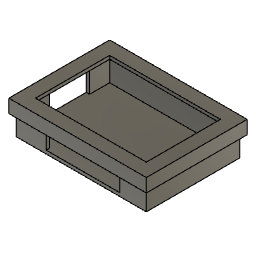
PCB box (Autodesk Fusion 360 design; units mm, degrees)
Autodesk Fusion 360 part; units mm, degrees
note: some values were not read from the file. Set by a fixed rule: which face or edge a step refers to.
sketch "Sketch1" plane through (0, 0, 0) normal (0, 0, 1) x (1, 0, 0) in component "base"
  line L0 (0, 0) -> (37, 0)
  line L1 (37, 0) -> (37, 26)
  line L2 (37, 26) -> (0, 26)
  line L3 (0, 26) -> (0, 0)
  dimension "d1" = 26
  dimension "d2" = 37
  constraint horizontal L0
  constraint vertical L1
  constraint horizontal L2
  constraint vertical L3
  constraint coincident L0.start L3.end
  measures "d1" distance of L0.end L1.end
  measures "d2" distance of L0.start L0.end
extrude "Extrude1" add sketch "Sketch1" along normal blind 8 makes body 1 in component "base"
shell "Shell1" thickness 1 outward yes removed faces 1 at (12.3333, 8.6667, 8) on bodies 1 in component "base"
sketch "Sketch2" plane through (0, 0, 8) normal (0, 0, 1) x (-1, 0, 0) in component "base"
  line L0 (0, -26) -> (-37, -26)
  line L1 (-37, -26) -> (-37, 0)
  line L2 (-37, 0) -> (0, 0)
  line L3 (0, 0) -> (0, -26)
  line L4 (1, -27) -> (1, 1)
  line L5 (1, 1) -> (-38, 1)
  line L6 (-38, 1) -> (-38, -27)
  line L7 (-38, -27) -> (1, -27)
  line L8 (1, -20) -> (0, -20)
  line L9 (0, -20) -> (0, -8)
  line L10 (0, -8) -> (1, -8)
  line L11 (1, -8) -> (1, -20)
  dimension "d6" = 8
  dimension "d7" = 6
  constraint horizontal L8
  constraint vertical L9
  constraint horizontal L10
  constraint vertical L11
  constraint coincident L3 L9.end
  constraint coincident L4 L8.start
  measures "d6" distance of L2 L10
  measures "d7" distance of L0 L8
extrude "Extrude2" cut sketch "Sketch2" against normal up to surface (8 mm away) contours L3 L4 L8 L9 L10 L11 bodies 1 in component "base"
sketch "Sketch3" plane through (0, 0, 8) normal (0, 0, 1) x (-1, 0, 0) in component "base"
  line L0 (0, -8) -> (1, -8)
  line L1 (1, -8) -> (1, 1)
  line L2 (1, 1) -> (-38, 1)
  line L3 (-38, 1) -> (-38, -27)
  line L4 (-38, -27) -> (1, -27)
  line L5 (1, -27) -> (1, -20)
  line L6 (1, -20) -> (0, -20)
  line L7 (0, -20) -> (0, -26)
  line L8 (0, -26) -> (-37, -26)
  line L9 (-37, -26) -> (-37, 0)
  line L10 (-37, 0) -> (0, 0)
  line L11 (0, 0) -> (0, -8)
  line L12 (-8, 0) -> (-30, 0)
  line L13 (-30, 0) -> (-30, 1)
  line L14 (-30, 1) -> (-8, 1)
  line L15 (-8, 1) -> (-8, 0)
  dimension "d10" = 7
  dimension "d11" = 8
  constraint horizontal L12
  constraint vertical L13
  constraint horizontal L14
  constraint vertical L15
  constraint coincident L2 L13.end
  constraint coincident L10 L12.start
  measures "d10" distance of L9 L13
  measures "d11" distance of L11 L15
extrude "Extrude3" cut sketch "Sketch3" against normal up to surface (8 mm away) contours L2 L10 L12 L13 L14 L15 bodies 1 in component "base"
sketch "Sketch1 (2)" plane through (0, 0, 8) normal (0, 0, 1) x (-1, 0, 0) in component "top"
  line L0 (-8, 1) -> (-8, 0)
  line L1 (-8, 0) -> (0, 0)
  line L2 (0, 0) -> (0, -8)
  line L3 (0, -8) -> (1, -8)
  line L4 (1, -8) -> (1, 1)
  line L5 (1, 1) -> (-8, 1)
  line L6 (2.1, -28.1) -> (-39.1, -28.1)
  line L7 (-39.1, -28.1) -> (-39.1, 2.1)
  line L8 (-39.1, 2.1) -> (2.1, 2.1)
  line L9 (2.1, 2.1) -> (2.1, -28.1)
  line L10 (-30, 0) -> (-30, 1)
  line L11 (-30, 1) -> (-38, 1)
  line L12 (-38, 1) -> (-38, -27)
  line L13 (-38, -27) -> (1, -27)
  line L14 (1, -27) -> (1, -20)
  line L15 (1, -20) -> (0, -20)
  line L16 (0, -20) -> (0, -26)
  line L17 (0, -26) -> (-37, -26)
  line L18 (-37, -26) -> (-37, 0)
  line L19 (-37, 0) -> (-30, 0)
  dimension "d14" = 1.1
  dimension "d15" = 1.1
  dimension "d16" = 1.1
  dimension "d17" = 1.1
  constraint horizontal L6
  constraint vertical L7
  constraint horizontal L8
  constraint vertical L9
  measures "d14" distance of L6 L13
  measures "d15" distance of L8 L11
  measures "d16" distance of L7 L12
  measures "d17" distance of L4 L9
extrude "Extrude1'" add sketch "Sketch1 (2)" along normal blind 1 and the other way blind 3 separate body contours L0 L1 L2 L3 L4 L5 | L6 L7 L8 L9 | L10 L11 L12 L13 L14 L15 L16 L17 L18 L19 makes body 2 in component "top"
shell "Shell1'" thickness 1 removed faces 1 at (25.3667, 18.0333, 5) on bodies 2 in component "top"
sketch "Sketch2 (2)" plane through (0, 0, 9) normal (0, 0, 1) x (-1, 0, 0) in component "top"
  line L0 (2.1, 2.1) -> (-39.1, 2.1)
  line L1 (-39.1, 2.1) -> (-39.1, -28.1)
  line L2 (-39.1, -28.1) -> (2.1, -28.1)
  line L3 (2.1, -28.1) -> (2.1, 2.1)
  line L4 (-1.9, -1.9) -> (-35.1, -1.9)
  line L5 (-35.1, -1.9) -> (-35.1, -24.1)
  line L6 (-35.1, -24.1) -> (-1.9, -24.1)
  line L7 (-1.9, -24.1) -> (-1.9, -1.9)
  dimension "d23" = -4
extrude "Extrude2'" cut sketch "Sketch2 (2)" against normal up to surface (1 mm away) contours L4 L5 L6 L7 bodies 2 in component "top"
component "base" placed x (1, 0, 0) y (0, 1, 0) z (0, 0, 1) at (0, 0, 0)
component "top" placed x (1, 0, 0) y (0, 1, 0) z (0, 0, 1) at (0, 0, 0)
